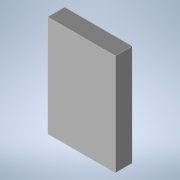
# Autodesk Inventor part: Foam_Hammer_Side
Saved by Autodesk Inventor 2021 (Build 250183000, 183)
## iProperties
Created: 2021-02-18
Part Number: Foam_Hammer_Side
Material: Polystyrene, Expanded
Document SubType Name: Modeling
Designer: negt20
Density: 0.05 g/cm^3
Appearance: Gray
Author: negt20
Autodesk Inventor part; units mm, degrees
ref_plane "YZ Plane" through (0, 0, 0) normal (1, 0, 0) x (0, 1, 0)
ref_plane "XZ Plane" through (0, 0, 0) normal (0, 1, 0) x (-1, 0, 0)
ref_plane "XY Plane" through (0, 0, 0) normal (0, 0, 1) x (1, 0, 0)
sketch "Sketch1" plane through (0, 0, 0) normal (0, 0, 1) x (1, 0, 0)
  line L0 (-50, 75) -> (50, 75)
  line L1 (50, 75) -> (50, -75)
  line L2 (50, -75) -> (-50, -75)
  line L3 (-50, -75) -> (-50, 75)
  point P0 (0, 0)
  point P1 (0, 75)
  point P2 (-50, 0)
  dimension "d0" = 100
  dimension "d1" = 150
  constraints: 8 end point, 2 midpoint, 2 parallel, 1 horizontal, 1 horizontal alignment, 1 perpendicular, 1 vertical alignment
  measures "d0" distance of L1.end L2.end
  measures "d1" distance of L0.end L1.end
extrude "Extrusion1" add sketch "Sketch1" along normal blind 25
sketch "Sketch2" plane through (0, 0, 25) normal (0, 0, 1) x (1, 0, 0)
  line L0 (-50, -75) -> (50, -75) projected
  line L1 (0, -75) -> (0, -50) construction
  line L2 (0, -50) -> (0, -40) construction
  line L3 (-5, 40) -> (5, 40) construction
  line L4 (5, 40) -> (5, -40)
  line L5 (5, -40) -> (-5, -40) construction
  line L6 (-5, -40) -> (-5, 40)
  arc A0 (-5, -40) -> (5, -40) centre (0, -40) ccw
  arc A1 (5, 40) -> (-5, 40) centre (0, 40) ccw
  line L7 (50, 75) -> (-50, 75) projected
  line L8 (0, 75) -> (0, 50) construction
  line L9 (0, 50) -> (0, 40) construction
  point P0 (0, 0)
  dimension "d4" = 25
  dimension "d5" = 10
  dimension "d6" = 10
  dimension "d8" = 25
  dimension "d11" = 10
  constraints: 16 end point, 4 midpoint, 4 point on circle, 3 coincident, 3 vertical, 2 centre point, 2 parallel, 1 horizontal, 1 perpendicular, 1 point on line
  measures "d4" distance of L1.start L1.end
  measures "d5" distance of L1.end L2.end
  measures "d6" distance of L4.end L5.end
  measures "d8" distance of L8.start L8.end
  measures "d11" distance of L8.end L9.end
extrude "Extrusion2" [suppressed]
body "Solid1"
